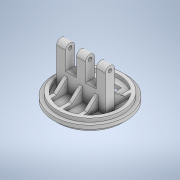
# Autodesk Inventor part: типа подшипник
Saved by Autodesk Inventor 2020.1 (Build 241239000, 239)
## iProperties
Created: 2022-04-03
Part Number: типа подшипник
Material: Типовые
Document SubType Name: Modeling
Designer: User
Density: 1 g/cm^3
Appearance: По умолчанию
Author: User
Autodesk Inventor part; units mm, degrees
ref_plane "YZ Plane" through (0, 0, 0) normal (1, 0, 0) x (0, 1, 0)
ref_plane "XZ Plane" through (0, 0, 0) normal (0, 1, 0) x (-1, 0, 0)
ref_plane "XY Plane" through (0, 0, 0) normal (0, 0, 1) x (1, 0, 0)
sketch "Эскиз1" plane through (0, 0, 0) normal (0, 1, 0) x (-1, 0, 0)
  circle A0 centre (0, 0) radius 40
  dimension "d0" = 80
  constraints: 1 centre point, 1 coincident
  measures "d0" diameter of A0
extrude "Выдавливание1" add sketch "Эскиз1" along normal blind 4
sketch "Эскиз2" plane through (0, 4, 0) normal (0, 1, 0) x (1, 0, 0)
  line L0 (-17, -10) -> (-27, -10)
  line L1 (-27, -10) -> (-27, 0)
  line L2 (-27, 0) -> (-17, 0)
  line L3 (-17, 0) -> (-17, -10)
  line L4 (27, -10) -> (17, -10)
  line L5 (17, -10) -> (17, 0)
  line L6 (17, 0) -> (27, 0)
  line L7 (27, 0) -> (27, -10)
  line L8 (5, -10) -> (-5, -10)
  line L9 (-5, -10) -> (-5, 0)
  line L10 (-5, 0) -> (5, 0)
  line L11 (5, 0) -> (5, -10)
  circle A0 centre (0, 0) radius 40 projected
  line L12 (0, 40) -> (0, 16.8758)
  line L13 (40, 0) -> (27.344, 0)
  line L14 (0, 0) -> (0, 40)
  line L15 (40, 0) -> (0, 0)
  line L16 (39.6863, -5) -> (-39.6863, -5)
  dimension "d3" = 10
  dimension "d4" = 12
  dimension "d5" = 10
  dimension "d14" = 5
  constraints: 34 end point, 6 horizontal, 6 parallel, 6 point on circle, 3 perpendicular, 2 equal length, 2 point on line, 2 vertical, 6 other
  measures "d3" distance of L6.end L4.start
  measures "d4" distance of L10.end L5.end
  measures "d5" distance of L9.end L10.end
  measures "d14" vertical distance of point (0, 0) L16.end
extrude "Выдавливание2" add sketch "Эскиз2" along normal blind 45 contours L0 L1 L16 L3 | L16 L1 L2 L3 | L16 L11 L8 L9 | L9 L10 L11 L16 | L16 L7 L4 L5 | L5 L6 L7 L16
sketch "Эскиз3" plane through (27, 4, 10) normal (1, 0, 0) x (0, 0, -1)
  line L0 (0, 45) -> (10, 45) projected
  line L1 (10, 0) -> (10, 45) projected
  circle A0 centre (5, 40) radius 2
  point P0 (10, -4)
  point P1 (5, 45)
  point P2 (10, 40)
  dimension "d8" = 5
  dimension "d9" = 4
  dimension "d20" = 0
  constraints: 1 centre point, 1 midpoint, 1 point on line
  measures "d8" distance of L0.end point (10, 40)
  measures "d9" diameter of A0
  measures "d20" vertical distance of point (10, 40) A0.centre
extrude "Выдавливание3" cut sketch "Эскиз3" against normal blind 100
fillet "Сопряжение1" radius 5 6 edges at (-22, 49, 10) (-22, 49, 0) (0, 49, 10) (0, 49, 0) (22, 49, 10) (22, 49, 0)
sketch "Эскиз4" plane through (0, 4, 0) normal (0, 1, 0) x (1, 0, 0)
  line L0 (10, 25) -> (-10, 25)
  line L1 (-10, 25) -> (-10, 5)
  line L2 (-10, 5) -> (10, 5)
  line L3 (10, 5) -> (10, 25)
  circle A0 centre (0, 0) radius 40 projected
  line L4 (0, 40) -> (0, 0)
  dimension "d15" = 20
  dimension "d16" = 20
  dimension "d17" = 5
  constraints: 10 end point, 2 parallel, 1 horizontal, 1 perpendicular, 1 vertical, 1 vertical alignment, 2 other
  measures "d15" distance of L0.end L1.end
  measures "d16" distance of L1.end L2.end
  measures "d17" vertical distance of L4.end L1.end
extrude "Выдавливание4" cut sketch "Эскиз4" against normal blind 10 contours L3 L2 L4 L0 | L4 L2 L1 L0
sketch "Эскиз5" plane through (0, 4, 0) normal (0, 1, 0) x (1, 0, 0)
  line L0 (-27, -10) -> (-27, 0) projected
  line L1 (17, 0) -> (27, 0) projected
  line L2 (-27, -10) -> (27, -10)
  line L3 (27, -10) -> (27, 0)
  line L4 (27, 0) -> (-27, 0)
  line L5 (-27, 0) -> (-27, -10)
  point P0 (0, 0)
  constraints: 8 end point, 2 parallel, 1 horizontal, 1 perpendicular
extrude "Выдавливание5" add sketch "Эскиз5" along normal blind 20
sketch "Эскиз6" plane through (0, 4, 0) normal (0, 1, 0) x (1, 0, 0)
  line L0 (-27, 0) -> (27, 0) projected
  line L1 (20, 0) -> (24, 0)
  line L2 (24, 0) -> (24, 20)
  line L3 (24, 20) -> (20, 20)
  line L4 (20, 20) -> (20, 0)
  line L5 (-24, 0) -> (-20, 0)
  line L6 (-20, 0) -> (-20, 20)
  line L7 (-20, 20) -> (-24, 20)
  line L8 (-24, 20) -> (-24, 0)
  line L9 (-5, -10) -> (5, -10) projected
  line L10 (-2, -10) -> (2, -10)
  line L11 (2, -10) -> (2, -30)
  line L12 (2, -30) -> (-2, -30)
  line L13 (-2, -30) -> (-2, -10)
  line L14 (-27, -10) -> (-17, -10) projected
  line L15 (-19, -10) -> (-15, -10)
  line L16 (-15, -10) -> (-15, -26)
  line L17 (-15, -26) -> (-19, -26)
  line L18 (-19, -26) -> (-19, -10)
  line L19 (27, -10) -> (-27, -10) projected
  line L20 (15, -10) -> (19, -10)
  line L21 (19, -10) -> (19, -26)
  line L22 (19, -26) -> (15, -26)
  line L23 (15, -26) -> (15, -10)
  line L24 (17, 0) -> (17, -10) projected
  line L25 (0, 0) -> (0, 4.7699)
  line L26 (-17, -10) -> (-17, 0) projected
  line L27 (-22, -10) -> (-22, 0)
  line L28 (17, -10) -> (27, -10) projected
  line L29 (22, -10) -> (22, 0)
  line L30 (-17, 0) -> (-27, 0) projected
  dimension "d23" = 4
  dimension "d24" = 20
  dimension "d25" = 16
  dimension "d26" = 20
  dimension "d27" = 0
  constraints: 46 end point, 15 parallel, 6 perpendicular, 5 horizontal, 5 point on line, 4 midpoint, 1 vertical, 8 other
  measures "d23" distance of L6.end L7.end
  measures "d24" distance of L12.end L10.start
  measures "d25" distance of L17.end L15.start
  measures "d26" distance of L7.end L5.start
  measures "d27" distance of L27.end point (-22, 0)
extrude "Выдавливание6" add sketch "Эскиз6" along normal blind 15 contours L8 L7 L6 L0 | L14 L15 L16 L17 L18 | L4 L3 L2 L0 | L19 L21 L22 L23 | L9 L11 L12 L13
sketch "Эскиз7" plane through (27, 4, 10) normal (1, 0, 0) x (0, 0, -1)
  line L0 (-16, 0) -> (0, 0) projected
  line L1 (-16, 0) -> (0, 15)
  line L2 (0, 0) -> (0, 30) projected
  line L3 (10, 0) -> (10, 30) projected
  line L4 (30, 0) -> (30, 15) projected
  line L5 (10, 15) -> (30, 0)
  line L6 (50, 0) -> (-30, 0) projected
  line L7 (-30, 0) -> (50, 0)
  line L8 (50, 0) -> (50, -10)
  line L9 (50, -10) -> (-30, -10)
  line L10 (-30, -10) -> (-30, 0)
  arc A0 (10, 40) -> (0, 40) centre (5, 40) ccw projected
  line L11 (10, 0) -> (5, 0)
  line L12 (5, 0) -> (5, 45)
  line L13 (5, 45) -> (10, 45)
  line L14 (10, 45) -> (10, 0)
  line L15 (5, 45) -> (0, 45)
  line L16 (0, 45) -> (0, 0)
  line L17 (0, 0) -> (5, 0)
  line L18 (5, 0) -> (5, 45)
  point P0 (10, -4)
  dimension "d32" = 0
  constraints: 28 end point, 6 parallel, 3 horizontal, 3 perpendicular, 2 midpoint, 1 point on circle
  measures "d32" distance of L6.start L7.end
extrude "Выдавливание7" cut sketch "Эскиз7" against normal mid plane 1000 keep common part
sketch "Эскиз8" plane through (0, 4, 0) normal (0, 1, 0) x (1, 0, 0)
  circle A0 centre (0, 0) radius 36
  circle A1 centre (0, 0) radius 40 projected
  circle A2 centre (0, 0) radius 32
  line L0 (-19, -10) -> (-15, -10) projected
  line L1 (-19, -10) -> (-15, -10)
  line L2 (-15, -10) -> (-15, -28.2666)
  line L3 (-15, -28.2666) -> (-19, -28.2666)
  line L4 (-19, -28.2666) -> (-19, -10)
  line L5 (19, -10) -> (19, -26) projected
  line L6 (19, -10) -> (15, -10)
  line L7 (15, -10) -> (15, -28.2666)
  line L8 (15, -28.2666) -> (19, -28.2666)
  line L9 (19, -28.2666) -> (19, -10)
  line L10 (-2, -26) -> (-2, -10) projected
  line L11 (-2, -10) -> (2, -10)
  line L12 (2, -10) -> (2, -36)
  line L13 (2, -36) -> (-2, -36)
  line L14 (-2, -36) -> (-2, -10)
  line L15 (20, 0) -> (20, 20) projected
  line L16 (20, 0) -> (24, 0)
  line L17 (24, 0) -> (24, 26.8328)
  line L18 (24, 26.8328) -> (20, 26.8328)
  line L19 (20, 26.8328) -> (20, 0)
  line L20 (-20, 0) -> (20, 0) projected
  line L21 (-20, 0) -> (-24, 0)
  line L22 (-24, 0) -> (-24, 26.8328)
  line L23 (-24, 26.8328) -> (-20, 26.8328)
  line L24 (-20, 26.8328) -> (-20, 0)
  point P0 (0, -40)
  point P1 (0, -36)
  point P2 (0, -32)
  point P3 (-20, 24.98)
  point P4 (-24, 21.166)
  point P5 (24, 21.166)
  point P6 (20, 24.98)
  point P7 (19, -25.7488)
  point P8 (-2, -31.9374)
  point P9 (2, -31.9374)
  point P10 (-19, -25.7488)
  dimension "d33" = 4
  dimension "d34" = 4
  constraints: 40 end point, 10 parallel, 6 point on circle, 5 horizontal, 5 perpendicular, 2 centre point, 2 coincident, 2 point on line, 1 vertical alignment, 1 other
  measures "d33" distance of A0.start point (0, -40)
  measures "d34" distance of A0.start A2.start
extrude "Выдавливание8" add sketch "Эскиз8" along normal blind 4 contours A0 L12 A2 L8 L9 L5 L17 | L18 L19 A2 L24 L23 A0 | L17 A2 L19 L18 | A0 L14 A2 L12 | L22 A2 L4 L3 L14 A0 | L23 L24 A2 L22 | L17 L16 L15 L19 A2 | A2 L14 L10 L11 L12 | A2 L24 L21 L22 | L7 L6 L5 A2 | A2 L5 L9 L8 | L4 L0 L2 A2 | A2 L3 L4
sketch "Эскиз9" plane through (0, 0, 0) normal (0, -1, 0) x (1, 0, 0)
  circle A0 centre (0, 0) radius 36
  circle A1 centre (0, 0) radius 32
  constraints: 2 centre point, 2 coincident
extrude "Выдавливание9" add sketch "Эскиз9" along normal blind 4
sketch "Эскиз10" plane through (0, 0, 0) normal (0, -1, 0) x (1, 0, 0)
  line L0 (-18.9031, -19.8094) -> (-14.76, -19.8094)
  line L1 (-14.76, -19.8094) -> (-14.76, -11.0052)
  line L2 (-14.76, -11.0052) -> (-18.9031, -11.0052)
  line L3 (-18.9031, -11.0052) -> (-18.9031, -19.8094)
  point P0 (0, 0)
  constraints: 8 end point, 2 parallel, 1 horizontal, 1 perpendicular
extrude "Выдавливание10" add sketch "Эскиз10" along normal blind 30
